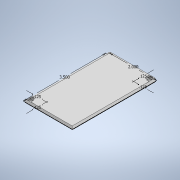
# Autodesk Inventor part: DualSensorReadout - Lid
Saved by Autodesk Inventor 2020 (Build 240168000, 168)
## iProperties
Created: 2024-01-28
Part Number: DualSensorReadout - Lid
Material: Generic
Document SubType Name: Modeling
Designer: Beaucage
Density: 1 g/cm^3
Appearance: Default
Author: Beaucage
Autodesk Inventor part; units mm, degrees
ref_plane "YZ Plane" through (0, 0, 0) normal (1, 0, 0) x (0, 1, 0)
ref_plane "XZ Plane" through (0, 0, 0) normal (0, 1, 0) x (-1, 0, 0)
ref_plane "XY Plane" through (0, 0, 0) normal (0, 0, 1) x (1, 0, 0)
sketch "Sketch1" plane through (0, 0, 0) normal (0, 1, 0) x (-1, 0, 0)
  line L0 (0, 0) -> (50.8, 0)
  line L1 (50.8, 0) -> (50.8, -88.9)
  line L2 (50.8, -88.9) -> (0, -88.9)
  line L3 (0, -88.9) -> (0, 0)
  line L4 (50.8, 0) -> (47.625, 0)
  line L5 (47.625, 0) -> (47.625, -3.175)
  line L6 (47.625, -3.175) -> (50.8, -3.175)
  line L7 (50.8, -3.175) -> (50.8, 0)
  line L8 (0, -88.9) -> (3.175, -88.9)
  line L9 (3.175, -88.9) -> (3.175, -85.725)
  line L10 (3.175, -85.725) -> (0, -85.725)
  line L11 (0, -85.725) -> (0, -88.9)
  dimension "d0" = 50.8
  dimension "d1" = 88.9
  dimension "d2" = 3.175
  dimension "d3" = 3.175
  dimension "d4" = 3.175
  dimension "d5" = 3.175
  constraints: 24 end point, 6 parallel, 3 horizontal, 3 perpendicular
  measures "d0" distance of L1.end L2.end
  measures "d1" distance of L0.end L1.end
  measures "d2" distance of L6.end L5.end
  measures "d3" distance of L5.end L4.end
  measures "d4" distance of L10.end L9.end
  measures "d5" distance of L9.end L8.end
extrude "Extrusion1" add sketch "Sketch1" along normal blind 3.175
sketch "Sketch2" plane through (0, 3.175, 0) normal (0, 1, 0) x (1, 0, 0)
  line L0 (-50.8, 0) -> (0, 0) projected
  line L1 (-50.8, 0) -> (-47.625, 0)
  line L2 (-47.625, 0) -> (-47.625, 3.175)
  line L3 (-47.625, 3.175) -> (-50.8, 3.175)
  line L4 (-50.8, 3.175) -> (-50.8, 0)
  line L5 (0, 88.9) -> (-50.8, 88.9) projected
  line L6 (0, 88.9) -> (-3.175, 88.9)
  line L7 (-3.175, 88.9) -> (-3.175, 85.725)
  line L8 (-3.175, 85.725) -> (0, 85.725)
  line L9 (0, 85.725) -> (0, 88.9)
  dimension "d15" = 3.175
  dimension "d16" = 3.175
  dimension "d17" = 3.175
  dimension "d18" = 3.175
  constraints: 16 end point, 4 parallel, 2 horizontal, 2 perpendicular
  measures "d15" distance of L3.end L2.end
  measures "d16" distance of L2.end L1.end
  measures "d17" distance of L8.end L7.end
  measures "d18" distance of L7.end L6.end
hole "Hole2" at (-47.625, 3.175, -3.175) at (-3.175, 3.175, -85.725) direction (0, -1, 0) diameter 3.2766 depth 7.9375 counterbore diameter 5.5626 counterbore depth 1.5875 clearance for "Socket Head Cap Screw" size "#4" standard "Ansi Unified Screw Threads"
fillet "Fillet1" radius 3.175 1 edges at (-50.8, 3.175, -44.45)
body "Solid1"
